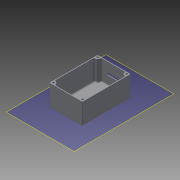
# Autodesk Inventor part: cuerpo
Saved by Autodesk Inventor 2015 (Build 190159000, 159)
## iProperties
Created: 2016-09-11
Part Number: cuerpo
Material: Generic
Document SubType Name: Modeling
Designer: Administrator
Density: 1 g/cm^3
Appearance: Default
Author: Administrator
Autodesk Inventor part; units mm, degrees
ref_plane "YZ Plane" through (0, 0, 0) normal (1, 0, 0) x (0, 1, 0)
ref_plane "XZ Plane" through (0, 0, 0) normal (0, 1, 0) x (-1, 0, 0)
ref_plane "XY Plane" through (0, 0, 0) normal (0, 0, 1) x (1, 0, 0)
sketch "Sketch1" plane through (0, 0, 0) normal (0, 0, 1) x (1, 0, 0)
  line L0 (-56, 0) -> (56, 0) projected
  line L1 (0, 81.9) -> (0, -81.9) projected
  line L2 (-40, 58.5) -> (40, 58.5)
  line L3 (40, 58.5) -> (40, -58.5)
  line L4 (40, -58.5) -> (-40, -58.5)
  line L5 (-40, -58.5) -> (-40, 58.5)
  line L6 (38.2, 56.7) -> (-38.2, 56.7)
  line L7 (-38.2, 56.7) -> (-38.2, -56.7)
  line L8 (-38.2, -56.7) -> (38.2, -56.7)
  line L9 (38.2, -56.7) -> (38.2, 56.7)
  point P0 (0, 0)
  dimension "d0" = 80
  dimension "d1" = 117
  dimension "d2" = 1.8
  constraints: 16 end point, 4 parallel, 2 perpendicular, 2 symmetric about line, 1 horizontal, 3 other
  measures "d0" distance of L2.start L2.end
  measures "d1" distance of L4.end L2.start
  measures "d2" distance between parallel lines of L2 L6
extrude "Extrusion1" add sketch "Sketch1" along normal blind 50 contours L5 L2 L1 L6 L7 L0 | L0 L7 L8 L1 L4 L5 | L1 L8 L9 L0 L3 L4 | L2 L3 L0 L9 L6 L1
ref_plane "Work Plane1" through (0, 0, -1.8) normal (0, 0, -1) x (-1, 0, 0)
sketch "Sketch2" plane through (0, 0, -1.8) normal (0, 0, -1) x (-1, 0, 0)
  line L0 (40, 58.5) -> (-40, 58.5) projected
  line L1 (-40, 58.5) -> (-40, -58.5) projected
  line L2 (-40, -58.5) -> (40, -58.5) projected
  line L3 (40, -58.5) -> (40, 58.5) projected
  point P0 (0, 0)
extrude "Extrusion2" add sketch "Sketch2" against normal blind 1.8
sketch "Sketch3" plane through (-40, 58.5, 50) normal (0, 1, 0) x (1, 0, 0)
  line L0 (0, 51.8) -> (0, 0) projected
  line L1 (80, 0) -> (0, 0) projected
  line L2 (80, 51.8) -> (80, 0) projected
  line L3 (0, 51.8) -> (80, 51.8) projected
  line L4 (0, 25.9) -> (185.6868, 25.9) construction
  line L5 (40, 0) -> (40, 25.9) construction
  line L6 (25, 28.9) -> (55, 28.9)
  line L7 (55, 28.9) -> (55, 22.9)
  line L8 (55, 22.9) -> (25, 22.9)
  line L9 (25, 22.9) -> (25, 28.9)
  point P0 (40, 50)
  dimension "d8" = 30
  dimension "d9" = 6
  constraints: 12 end point, 2 horizontal, 2 midpoint, 2 parallel, 2 perpendicular, 2 symmetric about line, 1 point on line
  measures "d8" distance of L6.start L6.end
  measures "d9" distance of L8.end L6.start
extrude "Extrusion3" cut sketch "Sketch3" against normal blind 2 contours L6 L7 L8 L9
sketch "Sketch4" plane through (0, 0, 0) normal (0, 0, 1) x (1, 0, 0)
  line L0 (38.2, -56.7) -> (38.2, 56.7) projected
  line L1 (38.2, 56.7) -> (-38.2, 56.7) projected
  line L2 (-38.2, 56.7) -> (-38.2, -56.7) projected
  line L3 (-38.2, -56.7) -> (38.2, -56.7) projected
  line L4 (40, 58.5) -> (-40, 58.5) projected
  line L5 (-40, 58.5) -> (-40, -58.5) projected
  line L6 (-58.4997, 0) -> (56.4166, 0) projected
  line L7 (0, -82.0878) -> (0, 83.0268) projected
  circle A0 centre (-35, 53.5) radius 5
  circle A1 centre (35, 53.5) radius 5
  circle A2 centre (-35, -53.5) radius 5
  circle A3 centre (35, -53.5) radius 5
  point P0 (0, 0)
  dimension "d14" = 10
  constraints: 4 centre point, 3 symmetric about line, 2 tangent, 3 other
  measures "d14" diameter of A0
extrude "Extrusion4" add sketch "Sketch4" along normal blind 50 contours L3 A3 L0 | L0 A3 L3 | A1 L1 L0 | L0 L1 A1 | A2 L2 L3 | L3 L2 A2 | A0 L1 L2 | L2 L1 A0
fillet "Fillet2" radius 4 8 edges at (31.1581, 56.7, 25) (38.2, 49.6581, 25) (-31.1581, 56.7, 25) (-38.2, 49.6581, 25) (-38.2, -49.6581, 25) (-31.1581, -56.7, 25) (31.1581, -56.7, 25) (38.2, -49.6581, 25)
sketch "Sketch5" plane through (0, 0, 50) normal (0, 0, 1) x (1, 0, 0)
  line L0 (40, -58.5) -> (40, 58.5) projected
  line L1 (40, 58.5) -> (-40, 58.5) projected
  line L2 (-40, 58.5) -> (-40, -58.5) projected
  line L3 (-40, -58.5) -> (40, -58.5) projected
  arc A0 (34.5556, -48.5198) -> (30.0198, -53.0556) centre (35, -53.5) ccw projected
  arc A1 (26.0356, -56.7) -> (30.0198, -53.0556) centre (26.0356, -52.7) ccw projected
  line L4 (26.0356, -56.7) -> (-26.0356, -56.7) projected
  arc A2 (-30.0198, -53.0556) -> (-26.0356, -56.7) centre (-26.0356, -52.7) ccw projected
  arc A3 (-30.0198, -53.0556) -> (-34.5556, -48.5198) centre (-35, -53.5) ccw projected
  arc A4 (-38.2, -44.5356) -> (-34.5556, -48.5198) centre (-34.2, -44.5356) ccw projected
  line L5 (-38.2, -44.5356) -> (-38.2, 44.5356) projected
  arc A5 (-34.5556, 48.5198) -> (-38.2, 44.5356) centre (-34.2, 44.5356) ccw projected
  arc A6 (-34.5556, 48.5198) -> (-30.0198, 53.0556) centre (-35, 53.5) ccw projected
  arc A7 (-26.0356, 56.7) -> (-30.0198, 53.0556) centre (-26.0356, 52.7) ccw projected
  line L6 (-26.0356, 56.7) -> (26.0356, 56.7) projected
  arc A8 (30.0198, 53.0556) -> (26.0356, 56.7) centre (26.0356, 52.7) ccw projected
  arc A9 (30.0198, 53.0556) -> (34.5556, 48.5198) centre (35, 53.5) ccw projected
  arc A10 (38.2, 44.5356) -> (34.5556, 48.5198) centre (34.2, 44.5356) ccw projected
  line L7 (38.2, 44.5356) -> (38.2, -44.5356) projected
  arc A11 (34.5556, -48.5198) -> (38.2, -44.5356) centre (34.2, -44.5356) ccw projected
  circle A12 centre (-35, 53.5) radius 2.1
  line L8 (-56, 0) -> (56, 0) projected
  line L9 (0, -81.9) -> (0, 81.9) projected
  circle A13 centre (35, 53.5) radius 2.1
  circle A14 centre (-35, -53.5) radius 2.1
  circle A15 centre (35, -53.5) radius 2.1
  point P0 (0, 0)
  dimension "d18" = 4.2
  constraints: 4 centre point, 3 symmetric about line, 1 coincident, 3 other
  measures "d18" diameter of A12
extrude "Extrusion5" add sketch "Sketch5" along normal blind 3 contours A12 | A13 | A14 | A15
fillet "Fillet3" radius 0.8 4 edges at (-37.1, 53.5, 50) (-37.1, -53.5, 50) (32.9, -53.5, 50) (32.9, 53.5, 50)
fillet "Fillet4" radius 2 8 edges at (-40, -58.5, 24.1) (0, -58.5, -1.8) (40, -58.5, 24.1) (-40, 0, -1.8) (0, 58.5, -1.8) (40, 58.5, 24.1) (-40, 58.5, 24.1) (40, 0, -1.8)
fillet "Fillet1" radius 3 4 edges at (-38.2, 0, 0) (0, 56.7, 0) (38.2, 0, 0) (0, -56.7, 0)
body "Solid1"
